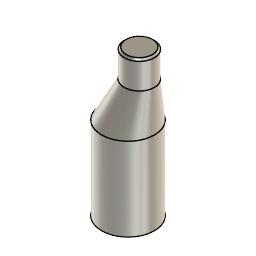
Input shaft_ (Autodesk Fusion 360 design; units mm, degrees)
Autodesk Fusion 360 part; units mm, degrees
sketch "Sketch1" plane through (0, 0, 0) normal (0, 0, 1) x (1, 0, 0)
  circle A0 centre (0, 0) radius 7
  line L0 (-2.1, -1.3565) -> (-2.1, 1.3565)
  arc A1 (-2.1, -1.3565) -> (-2.1, 1.3565) centre (0, 0) ccw
  dimension "d1" = 14
  dimension "d8" = 5
  dimension "d9" = 2.1
  constraint coincident A0.centre A1.centre
  constraint concentric A0 A1
  constraint vertical L0
  measures "d1" diameter of A0
  measures "d8" diameter of A1
  measures "d9" distance of A0.centre L0
extrude "Extrude1" add sketch "Sketch1" along normal blind 22 contours A0 | L0 A1 makes body 1
ref_plane "WorkPlane1" through (0, 0, 40.2) normal (0, 0, 1) x (1, 0, 0)
sketch "Sketch2" plane through (0, 0, 40.2) normal (0, 0, 1) x (1, 0, 0)
  circle A0 centre (0, 0) radius 7
  circle A1 centre (3, 0) radius 4
  dimension "d5" = 8
  constraint horizontal A0.centre A1.centre
  constraint tangent A0 A1
  measures "d5" diameter of A1
extrude "Extrude2" add sketch "Sketch2" against normal blind 7.3 separate body contours A1 makes body 2
loft "Loft1" add section 1 face at (3.1171, 1.096, 32.9) section 2 face at (1.11, -1.8763, 22) on bodies 1 2 bodies 1 2
extrude "Extrude3" cut sketch "Sketch1" along normal blind 21 contours L0 A1 bodies 1
chamfer "Chamfer1" distance 0.5 angle 45 1 edges at (-0.7293, -1.4465, 40.2) on bodies 1 2
